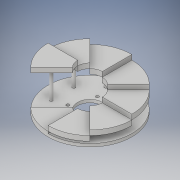
# Autodesk Inventor part: DesnivelSharp
Saved by Autodesk Inventor 2019 (Build 230136000, 136)
## iProperties
Created: 2019-12-22
Part Number: DesnivelSharp
Material: Generic
Document SubType Name: Modeling
Designer: Sergio
Density: 1 g/cm^3
Appearance: Default
Author: Sergio
Autodesk Inventor part; units mm, degrees
ref_plane "YZ Plane" through (0, 0, 0) normal (1, 0, 0) x (0, 1, 0)
ref_plane "XZ Plane" through (0, 0, 0) normal (0, 1, 0) x (-1, 0, 0)
ref_plane "XY Plane" through (0, 0, 0) normal (0, 0, 1) x (1, 0, 0)
sketch "Sketch1" plane through (0, 0, 0) normal (0, 1, 0) x (-1, 0, 0)
  circle A0 centre (0, 0) radius 12.5
  circle A1 centre (0, 0) radius 42.5
  line L0 (-8.8388, 8.8388) -> (-30.052, 30.052)
  line L1 (8.8388, -8.8388) -> (30.052, -30.052)
  line L2 (8.8388, 8.8388) -> (30.052, 30.052)
  line L3 (-8.8388, -8.8388) -> (-30.052, -30.052)
  line L4 (0, 42.5) -> (0, 12.5)
  line L5 (0, -12.5) -> (0, -42.5)
  line L6 (42.5, 0) -> (12.5, 0)
  line L7 (-12.5, 0) -> (-42.5, 0)
  dimension "d0" = 25
  dimension "d2" = 30
  constraints: 16 end point, 4 perpendicular, 2 coincident, 2 horizontal, 1 point on line, 20 other
extrude "Extrusion1" add sketch "Sketch1" along normal blind 5 contours A0 L4 A1 L2
sketch "Sketch2" plane through (0, 0, 0) normal (0, 1, 0) x (-1, 0, 0)
  circle A0 centre (0, 0) radius 12.5
  circle A1 centre (0, 0) radius 42.5
  line L0 (-8.8388, 8.8388) -> (-30.052, 30.052)
  line L1 (8.8388, -8.8388) -> (30.052, -30.052)
  line L2 (8.8388, 8.8388) -> (30.052, 30.052)
  line L3 (-8.8388, -8.8388) -> (-30.052, -30.052)
  line L4 (0, 42.5) -> (0, 12.5)
  line L5 (0, -12.5) -> (0, -42.5)
  line L6 (42.5, 0) -> (12.5, 0)
  line L7 (-12.5, 0) -> (-42.5, 0)
  dimension "d7" = 25
  dimension "d8" = 30
  constraints: 16 end point, 4 perpendicular, 2 coincident, 2 horizontal, 1 point on line, 20 other
extrude "Extrusion2" add sketch "Sketch2" along normal blind 10 contours A0 L0 A1 L4
sketch "Sketch3" plane through (0, 0, 0) normal (0, 1, 0) x (-1, 0, 0)
  circle A0 centre (0, 0) radius 12.5
  circle A1 centre (0, 0) radius 42.5
  line L0 (-8.8388, 8.8388) -> (-30.052, 30.052)
  line L1 (8.8388, -8.8388) -> (30.052, -30.052)
  line L2 (8.8388, 8.8388) -> (30.052, 30.052)
  line L3 (-8.8388, -8.8388) -> (-30.052, -30.052)
  line L4 (0, 42.5) -> (0, 12.5)
  line L5 (0, -12.5) -> (0, -42.5)
  line L6 (42.5, 0) -> (12.5, 0)
  line L7 (-12.5, 0) -> (-42.5, 0)
  dimension "d11" = 25
  dimension "d12" = 30
  constraints: 16 end point, 4 perpendicular, 2 coincident, 2 horizontal, 1 point on line, 20 other
extrude "Extrusion3" add sketch "Sketch3" along normal blind 15 contours A0 L7 A1 L0
sketch "Sketch4" plane through (0, 0, 0) normal (0, 1, 0) x (-1, 0, 0)
  circle A0 centre (0, 0) radius 12.5
  circle A1 centre (0, 0) radius 42.5
  line L0 (-8.8388, 8.8388) -> (-30.052, 30.052)
  line L1 (8.8388, -8.8388) -> (30.052, -30.052)
  line L2 (8.8388, 8.8388) -> (30.052, 30.052)
  line L3 (-8.8388, -8.8388) -> (-30.052, -30.052)
  line L4 (0, 42.5) -> (0, 12.5)
  line L5 (0, -12.5) -> (0, -42.5)
  line L6 (42.5, 0) -> (12.5, 0)
  line L7 (-12.5, 0) -> (-42.5, 0)
  dimension "d15" = 25
  dimension "d16" = 30
  constraints: 16 end point, 4 perpendicular, 2 coincident, 2 horizontal, 1 point on line, 20 other
extrude "Extrusion4" add sketch "Sketch4" along normal blind 20 contours L3 A1 L7 A0
sketch "Sketch8" plane through (0, 0, 0) normal (0, 1, 0) x (-1, 0, 0)
  circle A0 centre (0, 0) radius 12.5
  circle A1 centre (0, 0) radius 42.5
  line L0 (-8.8388, 8.8388) -> (-30.052, 30.052)
  line L1 (8.8388, -8.8388) -> (30.052, -30.052)
  line L2 (8.8388, 8.8388) -> (30.052, 30.052)
  line L3 (-8.8388, -8.8388) -> (-30.052, -30.052)
  line L4 (0, 42.5) -> (0, 12.5)
  line L5 (0, -12.5) -> (0, -42.5)
  line L6 (42.5, 0) -> (12.5, 0)
  line L7 (-12.5, 0) -> (-42.5, 0)
  dimension "d31" = 25
  dimension "d32" = 30
  constraints: 16 end point, 4 perpendicular, 2 coincident, 2 horizontal, 1 point on line, 20 other
extrude "Extrusion8" add sketch "Sketch8" along normal blind 25 contours L5 A1 L3 A0
sketch "Sketch7" plane through (0, 0, 0) normal (0, 1, 0) x (-1, 0, 0)
  circle A0 centre (0, 0) radius 12.5
  circle A1 centre (0, 0) radius 42.5
  line L0 (-8.8388, 8.8388) -> (-30.052, 30.052)
  line L1 (8.8388, -8.8388) -> (30.052, -30.052)
  line L2 (8.8388, 8.8388) -> (30.052, 30.052)
  line L3 (-8.8388, -8.8388) -> (-30.052, -30.052)
  line L4 (0, 42.5) -> (0, 12.5)
  line L5 (0, -12.5) -> (0, -42.5)
  line L6 (42.5, 0) -> (12.5, 0)
  line L7 (-12.5, 0) -> (-42.5, 0)
  dimension "d27" = 25
  dimension "d28" = 30
  constraints: 16 end point, 4 perpendicular, 2 coincident, 2 horizontal, 1 point on line, 20 other
extrude "Extrusion7" add sketch "Sketch7" along normal blind 30 contours L1 A1 L5 A0
sketch "Sketch6" plane through (0, 0, 0) normal (0, 1, 0) x (-1, 0, 0)
  circle A0 centre (0, 0) radius 12.5
  circle A1 centre (0, 0) radius 42.5
  line L0 (-8.8388, 8.8388) -> (-30.052, 30.052)
  line L1 (8.8388, -8.8388) -> (30.052, -30.052)
  line L2 (8.8388, 8.8388) -> (30.052, 30.052)
  line L3 (-8.8388, -8.8388) -> (-30.052, -30.052)
  line L4 (0, 42.5) -> (0, 12.5)
  line L5 (0, -12.5) -> (0, -42.5)
  line L6 (42.5, 0) -> (12.5, 0)
  line L7 (-12.5, 0) -> (-42.5, 0)
  dimension "d23" = 25
  dimension "d24" = 30
  constraints: 16 end point, 4 perpendicular, 2 coincident, 2 horizontal, 1 point on line, 20 other
extrude "Extrusion6" add sketch "Sketch6" along normal blind 35 contours L6 A1 L1 A0
sketch "Sketch5" plane through (0, 0, 0) normal (0, 1, 0) x (-1, 0, 0)
  circle A0 centre (0, 0) radius 12.5
  circle A1 centre (0, 0) radius 42.5
  line L0 (-8.8388, 8.8388) -> (-30.052, 30.052)
  line L1 (8.8388, -8.8388) -> (30.052, -30.052)
  line L2 (8.8388, 8.8388) -> (30.052, 30.052)
  line L3 (-8.8388, -8.8388) -> (-30.052, -30.052)
  line L4 (0, 42.5) -> (0, 12.5)
  line L5 (0, -12.5) -> (0, -42.5)
  line L6 (42.5, 0) -> (12.5, 0)
  line L7 (-12.5, 0) -> (-42.5, 0)
  dimension "d19" = 25
  dimension "d20" = 30
  constraints: 16 end point, 4 perpendicular, 2 coincident, 2 horizontal, 1 point on line, 20 other
extrude "Extrusion5" add sketch "Sketch5" along normal blind 40 contours A0 L2 A1 L6
sketch "Sketch9" plane through (0, 0, 0) normal (0, -1, 0) x (1, 0, 0)
  circle A0 centre (0, 0) radius 12.5
  circle A1 centre (0, 0) radius 42.5
  line L0 (-8.8388, 8.8388) -> (-30.052, 30.052)
  line L1 (8.8388, -8.8388) -> (30.052, -30.052)
  line L2 (8.8388, 8.8388) -> (30.052, 30.052)
  line L3 (-8.8388, -8.8388) -> (-30.052, -30.052)
  line L4 (0, 42.5) -> (0, 12.5)
  line L5 (0, -12.5) -> (0, -42.5)
  line L6 (42.5, 0) -> (12.5, 0)
  line L7 (-12.5, 0) -> (-42.5, 0)
  circle A2 centre (-11.3809, 27.7772) radius 1.5
  circle A3 centre (-27.6889, 11.5939) radius 1.5
  circle A4 centre (-27.7772, -11.3809) radius 1.5
  circle A5 centre (-11.5939, -27.6889) radius 1.5
  circle A6 centre (11.3809, -27.7772) radius 1.5
  circle A7 centre (27.6889, -11.5939) radius 1.5
  circle A8 centre (27.7772, 11.3809) radius 1.5
  circle A9 centre (11.5939, 27.6889) radius 1.5
  arc A10 (0, 42.5) -> (-30.052, 30.052) centre (0, 0) ccw projected
  line L8 (0, 0) -> (-21.5472, 0) construction
  line L9 (0, 0) -> (-13.7699, 33.608) construction
  dimension "d38" = 25
  dimension "d39" = 30
  dimension "d40" = 3
  dimension "d43" = 360
  constraints: 20 end point, 8 centre point, 4 perpendicular, 3 point on line, 2 coincident, 2 horizontal, 37 other
  measures "d40" diameter of A2
extrude "Extrusion9" cut sketch "Sketch9" against normal blind 35 contours A0 L7 A1 L0
sketch "Sketch10" plane through (0, 0, 0) normal (0, -1, 0) x (1, 0, 0)
  circle A0 centre (0, 0) radius 12.5
  circle A1 centre (0, 0) radius 42.5
  line L0 (-8.8388, 8.8388) -> (-30.052, 30.052)
  line L1 (8.8388, -8.8388) -> (30.052, -30.052)
  line L2 (8.8388, 8.8388) -> (30.052, 30.052)
  line L3 (-8.8388, -8.8388) -> (-30.052, -30.052)
  line L4 (0, 42.5) -> (0, 12.5)
  line L5 (0, -12.5) -> (0, -42.5)
  line L6 (42.5, 0) -> (12.5, 0)
  line L7 (-12.5, 0) -> (-42.5, 0)
  circle A2 centre (-11.3809, 27.7772) radius 1.5
  circle A3 centre (-27.6889, 11.5939) radius 1.5
  circle A4 centre (-27.7772, -11.3809) radius 1.5
  circle A5 centre (-11.5939, -27.6889) radius 1.5
  circle A6 centre (11.3809, -27.7772) radius 1.5
  circle A7 centre (27.6889, -11.5939) radius 1.5
  circle A8 centre (27.7772, 11.3809) radius 1.5
  circle A9 centre (11.5939, 27.6889) radius 1.5
  arc A10 (0, 42.5) -> (-30.052, 30.052) centre (0, 0) ccw
  line L8 (0, 0) -> (-21.5472, 0) construction
  line L9 (0, 0) -> (-13.7699, 33.608) construction
  dimension "d52" = 25
  dimension "d53" = 30
  dimension "d54" = 3
  dimension "d55" = 360
  constraints: 20 end point, 9 centre point, 4 perpendicular, 3 point on line, 2 coincident, 2 horizontal, 2 point on circle, 37 other
  measures "d54" diameter of A2
extrude "Extrusion10" cut sketch "Sketch10" against normal blind 30 contours L3 A1 L7 A0
sketch "Sketch11" plane through (0, 0, 0) normal (0, -1, 0) x (1, 0, 0)
  circle A0 centre (0, 0) radius 12.5
  circle A1 centre (0, 0) radius 42.5
  line L0 (-8.8388, 8.8388) -> (-30.052, 30.052)
  line L1 (8.8388, -8.8388) -> (30.052, -30.052)
  line L2 (8.8388, 8.8388) -> (30.052, 30.052)
  line L3 (-8.8388, -8.8388) -> (-30.052, -30.052)
  line L4 (0, 42.5) -> (0, 12.5)
  line L5 (0, -12.5) -> (0, -42.5)
  line L6 (42.5, 0) -> (12.5, 0)
  line L7 (-12.5, 0) -> (-42.5, 0)
  circle A2 centre (-11.3809, 27.7772) radius 1.5
  circle A3 centre (-27.6889, 11.5939) radius 1.5
  circle A4 centre (-27.7772, -11.3809) radius 1.5
  circle A5 centre (-11.5939, -27.6889) radius 1.5
  circle A6 centre (11.3809, -27.7772) radius 1.5
  circle A7 centre (27.6889, -11.5939) radius 1.5
  circle A8 centre (27.7772, 11.3809) radius 1.5
  circle A9 centre (11.5939, 27.6889) radius 1.5
  arc A10 (0, 42.5) -> (-30.052, 30.052) centre (0, 0) ccw
  line L8 (0, 0) -> (-21.5472, 0) construction
  line L9 (0, 0) -> (-13.7699, 33.608) construction
  dimension "d60" = 25
  dimension "d61" = 30
  dimension "d62" = 3
  dimension "d63" = 360
  constraints: 20 end point, 9 centre point, 4 perpendicular, 3 point on line, 2 coincident, 2 horizontal, 2 point on circle, 37 other
  measures "d62" diameter of A2
extrude "Extrusion11" cut sketch "Sketch11" against normal blind 25 contours L5 A1 L3 A0
sketch "Sketch12" plane through (0, 0, 0) normal (0, -1, 0) x (1, 0, 0)
  circle A0 centre (0, 0) radius 12.5
  circle A1 centre (0, 0) radius 42.5
  line L0 (-8.8388, 8.8388) -> (-30.052, 30.052)
  line L1 (8.8388, -8.8388) -> (30.052, -30.052)
  line L2 (8.8388, 8.8388) -> (30.052, 30.052)
  line L3 (-8.8388, -8.8388) -> (-30.052, -30.052)
  line L4 (0, 42.5) -> (0, 12.5)
  line L5 (0, -12.5) -> (0, -42.5)
  line L6 (42.5, 0) -> (12.5, 0)
  line L7 (-12.5, 0) -> (-42.5, 0)
  circle A2 centre (-11.3809, 27.7772) radius 1.5
  circle A3 centre (-27.6889, 11.5939) radius 1.5
  circle A4 centre (-27.7772, -11.3809) radius 1.5
  circle A5 centre (-11.5939, -27.6889) radius 1.5
  circle A6 centre (11.3809, -27.7772) radius 1.5
  circle A7 centre (27.6889, -11.5939) radius 1.5
  circle A8 centre (27.7772, 11.3809) radius 1.5
  circle A9 centre (11.5939, 27.6889) radius 1.5
  arc A10 (0, 42.5) -> (-30.052, 30.052) centre (0, 0) ccw
  line L8 (0, 0) -> (-21.5472, 0) construction
  line L9 (0, 0) -> (-13.7699, 33.608) construction
  dimension "d68" = 25
  dimension "d69" = 30
  dimension "d70" = 3
  dimension "d71" = 360
  constraints: 20 end point, 9 centre point, 4 perpendicular, 3 point on line, 2 coincident, 2 horizontal, 2 point on circle, 37 other
  measures "d70" diameter of A2
extrude "Extrusion12" cut sketch "Sketch12" against normal blind 20 contours L1 A1 L5 A0
sketch "Sketch13" plane through (0, 0, 0) normal (0, -1, 0) x (1, 0, 0)
  circle A0 centre (0, 0) radius 12.5
  circle A1 centre (0, 0) radius 42.5
  line L0 (-8.8388, 8.8388) -> (-30.052, 30.052)
  line L1 (8.8388, -8.8388) -> (30.052, -30.052)
  line L2 (8.8388, 8.8388) -> (30.052, 30.052)
  line L3 (-8.8388, -8.8388) -> (-30.052, -30.052)
  line L4 (0, 42.5) -> (0, 12.5)
  line L5 (0, -12.5) -> (0, -42.5)
  line L6 (42.5, 0) -> (12.5, 0)
  line L7 (-12.5, 0) -> (-42.5, 0)
  circle A2 centre (-11.3809, 27.7772) radius 1.5
  circle A3 centre (-27.6889, 11.5939) radius 1.5
  circle A4 centre (-27.7772, -11.3809) radius 1.5
  circle A5 centre (-11.5939, -27.6889) radius 1.5
  circle A6 centre (11.3809, -27.7772) radius 1.5
  circle A7 centre (27.6889, -11.5939) radius 1.5
  circle A8 centre (27.7772, 11.3809) radius 1.5
  circle A9 centre (11.5939, 27.6889) radius 1.5
  arc A10 (0, 42.5) -> (-30.052, 30.052) centre (0, 0) ccw
  line L8 (0, 0) -> (-21.5472, 0) construction
  line L9 (0, 0) -> (-13.7699, 33.608) construction
  dimension "d76" = 25
  dimension "d77" = 30
  dimension "d78" = 3
  dimension "d79" = 360
  constraints: 20 end point, 9 centre point, 4 perpendicular, 3 point on line, 2 coincident, 2 horizontal, 2 point on circle, 37 other
  measures "d78" diameter of A2
extrude "Extrusion13" cut sketch "Sketch13" against normal blind 15 contours L6 A1 L1 A0
sketch "Sketch14" plane through (0, 0, 0) normal (0, -1, 0) x (1, 0, 0)
  circle A0 centre (0, 0) radius 12.5
  circle A1 centre (0, 0) radius 42.5
  line L0 (-8.8388, 8.8388) -> (-30.052, 30.052)
  line L1 (8.8388, -8.8388) -> (30.052, -30.052)
  line L2 (8.8388, 8.8388) -> (30.052, 30.052)
  line L3 (-8.8388, -8.8388) -> (-30.052, -30.052)
  line L4 (0, 42.5) -> (0, 12.5)
  line L5 (0, -12.5) -> (0, -42.5)
  line L6 (42.5, 0) -> (12.5, 0)
  line L7 (-12.5, 0) -> (-42.5, 0)
  circle A2 centre (-11.3809, 27.7772) radius 1.5
  circle A3 centre (-27.6889, 11.5939) radius 1.5
  circle A4 centre (-27.7772, -11.3809) radius 1.5
  circle A5 centre (-11.5939, -27.6889) radius 1.5
  circle A6 centre (11.3809, -27.7772) radius 1.5
  circle A7 centre (27.6889, -11.5939) radius 1.5
  circle A8 centre (27.7772, 11.3809) radius 1.5
  circle A9 centre (11.5939, 27.6889) radius 1.5
  arc A10 (0, 42.5) -> (-30.052, 30.052) centre (0, 0) ccw
  line L8 (0, 0) -> (-21.5472, 0) construction
  line L9 (0, 0) -> (-13.7699, 33.608) construction
  dimension "d84" = 25
  dimension "d85" = 30
  dimension "d86" = 3
  dimension "d87" = 360
  constraints: 20 end point, 9 centre point, 4 perpendicular, 3 point on line, 2 coincident, 2 horizontal, 2 point on circle, 37 other
  measures "d86" diameter of A2
extrude "Extrusion14" cut sketch "Sketch14" against normal blind 10 contours A0 L2 A1 L6
sketch "Sketch15" plane through (0, 0, 0) normal (0, -1, 0) x (1, 0, 0)
  circle A0 centre (0, 0) radius 12.5
  circle A1 centre (0, 0) radius 42.5
  line L0 (-8.8388, 8.8388) -> (-30.052, 30.052)
  line L1 (8.8388, -8.8388) -> (30.052, -30.052)
  line L2 (8.8388, 8.8388) -> (30.052, 30.052)
  line L3 (-8.8388, -8.8388) -> (-30.052, -30.052)
  line L4 (0, 42.5) -> (0, 12.5)
  line L5 (0, -12.5) -> (0, -42.5)
  line L6 (42.5, 0) -> (12.5, 0)
  line L7 (-12.5, 0) -> (-42.5, 0)
  circle A2 centre (-11.3809, 27.7772) radius 1.5
  circle A3 centre (-27.6889, 11.5939) radius 1.5
  circle A4 centre (-27.7772, -11.3809) radius 1.5
  circle A5 centre (-11.5939, -27.6889) radius 1.5
  circle A6 centre (11.3809, -27.7772) radius 1.5
  circle A7 centre (27.6889, -11.5939) radius 1.5
  circle A8 centre (27.7772, 11.3809) radius 1.5
  circle A9 centre (11.5939, 27.6889) radius 1.5
  arc A10 (0, 42.5) -> (-30.052, 30.052) centre (0, 0) ccw
  line L8 (0, 0) -> (-21.5472, 0) construction
  line L9 (0, 0) -> (-13.7699, 33.608) construction
  dimension "d92" = 25
  dimension "d93" = 30
  dimension "d94" = 3
  dimension "d95" = 360
  constraints: 20 end point, 9 centre point, 4 perpendicular, 3 point on line, 2 coincident, 2 horizontal, 2 point on circle, 37 other
  measures "d94" diameter of A2
extrude "Extrusion15" cut sketch "Sketch15" against normal blind 5 contours A0 L4 A1 L2
sketch "Sketch18" plane through (0, 0, 0) normal (0, 1, 0) x (-1, 0, 0)
  circle A0 centre (0, 0) radius 42.5
  circle A1 centre (0, 0) radius 12.5
  dimension "d105" = 85
  dimension "d106" = 25
  constraints: 2 centre point, 2 coincident
  measures "d105" diameter of A0
  measures "d106" diameter of A1
extrude "Extrusion18" add sketch "Sketch18" along normal blind 3
sketch "Sketch19" plane through (0, 0, 0) normal (0, -1, 0) x (1, 0, 0)
  circle A0 centre (0, 0) radius 16.75
  circle A1 centre (14.9821, -7.4899) radius 1.5
  circle A2 centre (0, 0) radius 12.5
  circle A3 centre (7.4899, 14.9821) radius 1.5
  circle A4 centre (-14.9821, 7.4899) radius 1.5
  circle A5 centre (-7.4899, -14.9821) radius 1.5
  dimension "d110" = 33.5
  dimension "d111" = 3
  dimension "d112" = 25
  dimension "d115" = 360
  constraints: 5 centre point, 2 coincident, 12 other
  measures "d111" diameter of A1
  measures "d112" diameter of A2
extrude "Extrusion19" cut sketch "Sketch19" against normal blind 5 contours A3 A0 | A0 A3 | A1 A0 | A0 A1 | A4 A0 | A0 A4 | A5 A0 | A0 A5
body "Solid1"
